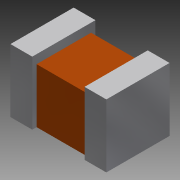
# Autodesk Inventor part: 0806Cap
Saved by Autodesk Inventor 2014 (Build 180170000, 170)
## iProperties
Created: 2015-11-06
Part Number: 0806Cap
Material: Generic
Document SubType Name: Modeling
Designer: Owner
Density: 1 g/cm^3
Appearance: Default
Author: Owner
Autodesk Inventor part; units mm, degrees
ref_plane "YZ Plane" through (0, 0, 0) normal (1, 0, 0) x (0, 1, 0)
ref_plane "XZ Plane" through (0, 0, 0) normal (0, 1, 0) x (-1, 0, 0)
ref_plane "XY Plane" through (0, 0, 0) normal (0, 0, 1) x (1, 0, 0)
sketch "Sketch1" plane through (0, 0, 0) normal (0, 1, 0) x (-1, 0, 0)
  line L0 (-0.8185, 0.4809) -> (1.1815, 0.4809)
  line L1 (1.1815, 0.4809) -> (1.1815, -0.7691)
  line L2 (1.1815, -0.7691) -> (-0.8185, -0.7691)
  line L3 (-0.8185, -0.7691) -> (-0.8185, 0.4809)
  point P0 (0, 0)
  dimension "d0" = 2
  dimension "d1" = 1.25
  constraints: 8 end point, 2 parallel, 1 horizontal, 1 perpendicular
  measures "d0" distance of L0.start L0.end
  measures "d1" distance of L0.end L1.end
extrude "Extrusion1" add sketch "Sketch1" along normal blind 1.25
sketch "Sketch2" plane through (0, 0, 0) normal (0, -1, 0) x (1, 0, 0)
  line L0 (0.8185, 0.4809) -> (-1.1815, 0.4809) projected
  line L1 (0.8185, -0.7691) -> (0.8185, 0.4809) projected
  line L2 (-1.2815, 0.5809) -> (-0.7815, 0.5809)
  line L3 (-0.7815, 0.5809) -> (-0.7815, -0.8691)
  line L4 (-0.7815, -0.8691) -> (-1.2815, -0.8691)
  line L5 (-1.2815, -0.8691) -> (-1.2815, 0.5809)
  line L6 (0.4185, 0.5809) -> (0.9185, 0.5809)
  line L7 (0.9185, 0.5809) -> (0.9185, -0.8691)
  line L8 (0.9185, -0.8691) -> (0.4185, -0.8691)
  line L9 (0.4185, -0.8691) -> (0.4185, 0.5809)
  point P0 (0, 0)
  dimension "d4" = 0.5
  dimension "d5" = 0.5
  dimension "d6" = 1.45
  dimension "d7" = 1.45
  dimension "d8" = 0.1
  dimension "d9" = 0.1
  dimension "d10" = 2.2
  dimension "d11" = 0.1
  constraints: 16 end point, 4 parallel, 2 horizontal, 2 perpendicular
  measures "d4" distance of L2.start L2.end
  measures "d5" distance of L6.start L6.end
  measures "d6" distance of L4.end L2.start
  measures "d7" distance of L6.end L7.end
  measures "d8" distance between parallel lines of L0 L2
  measures "d9" distance between parallel lines of L0 L6
  measures "d10" distance between parallel lines of L7 L5
  measures "d11" distance between parallel lines of L1 L7
extrude "Extrusion2" add sketch "Sketch2" against normal blind 1.45
body "Solid1"
